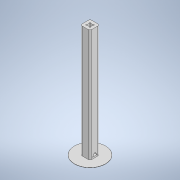
# Autodesk Inventor part: 130mm Rod Template
Saved by Autodesk Inventor 2022 (Build 260153000, 153)
## iProperties
Created: 2022-06-07
Part Number: 130mm Rod Template
Material: Generic
Document SubType Name: Modeling
Designer: Nick
Density: 1 g/cm^3
Appearance: Default
Author: Nick
Autodesk Inventor part; units mm, degrees
ref_plane "YZ Plane" through (0, 0, 0) normal (1, 0, 0) x (0, 1, 0)
ref_plane "XZ Plane" through (0, 0, 0) normal (0, 1, 0) x (-1, 0, 0)
ref_plane "XY Plane" through (0, 0, 0) normal (0, 0, 1) x (1, 0, 0)
sketch "Sketch1" plane through (0, 0, 0) normal (0, 1, 0) x (-1, 0, 0)
  circle A0 centre (0, 0) radius 2
  arc A1 (2.5, 2.1794) -> (2.5, -2.1794) centre (7, 0) ccw
  arc A2 (2.1794, -2.5) -> (-2.1794, -2.5) centre (0, -7) ccw
  arc A3 (-2.5, -2.1794) -> (-2.5, 2.1794) centre (-7, 0) ccw
  arc A4 (-2.1794, 2.5) -> (2.1794, 2.5) centre (0, 7) ccw
  line L0 (2.5, 2.5) -> (-2.5, 2.5)
  line L1 (-2.5, 2.5) -> (-2.5, -2.5)
  line L2 (-2.5, -2.5) -> (2.5, -2.5)
  line L3 (2.5, -2.5) -> (2.5, 2.5)
  line L4 (-5.5, -5.5) -> (-5.5, 5.5)
  line L5 (-5.5, 5.5) -> (5.5, 5.5)
  line L6 (5.5, 5.5) -> (5.5, -5.5)
  line L7 (5.5, -5.5) -> (-5.5, -5.5)
  point P0 (2.5, 0)
  point P1 (0, -2.5)
  dimension "d0" = 4
  dimension "d1" = 5
  dimension "d2" = 5
  dimension "d3" = 3
  constraints: 16 end point, 8 point on circle, 8 point on line, 5 centre point, 4 parallel, 4 tangent, 3 equal radius, 3 horizontal alignment, 3 perpendicular, 3 vertical alignment, 2 midpoint, 1 coincident, 1 horizontal, 3 other
  measures "d0" diameter of A0
  measures "d1" distance of L0.start L0.end
  measures "d2" radius of A4
  measures "d3" distance between parallel lines of L1 L4
extrude "Extrusion1" add sketch "Sketch1" along normal blind 125 contours A1 L3 | A4 L0 | A2 L2 | A3 L1 | L4 L5 L6 L7
sketch "Sketch2" plane through (5.5, 0, -5.5) normal (0, 0, -1) x (-1, 0, 0)
  line L0 (11, 125) -> (11, 0) construction
  line L1 (11, 0) -> (0, 0) construction
  line L2 (0, 0) -> (0, 125) construction
  line L3 (0, 125) -> (11, 125) construction
  line L4 (0, 0) -> (0, 125) projected
  line L5 (0, 125) -> (11, 125) projected
  line L6 (11, 0) -> (11, 125) projected
  line L7 (0, 0) -> (11, 0) projected
  line L8 (2.45, 72.5101) -> (2.45, 75.486)
  line L9 (2.45, 75.486) -> (3.0729, 75.486)
  line L10 (3.0729, 75.486) -> (3.0729, 74.3787)
  line L11 (3.0729, 74.3787) -> (7.1609, 74.3787)
  line L12 (7.1609, 74.3787) -> (7.1609, 75.486)
  line L13 (7.1609, 75.486) -> (7.7195, 75.486)
  spline S0 degree 2 poles (7.7195, 75.486) (7.7195, 74.8582) (8.0754, 74.265) (8.5698, 74.2254) knots 0 0 0 1 2 2 2
  line L14 (8.5698, 74.2254) -> (8.5698, 73.5927)
  line L15 (8.5698, 73.5927) -> (3.0729, 73.5927)
  line L16 (3.0729, 73.5927) -> (3.0729, 72.5101)
  line L17 (3.0729, 72.5101) -> (2.45, 72.5101)
  spline S1 degree 2 poles (7.9716, 69.7419) (7.9716, 69.9643) (7.8629, 70.4043) (7.7788, 70.6169) knots 0 0 0 1 2 2 2
  spline S2 degree 2 poles (7.7788, 70.6169) (7.6948, 70.8146) (7.5169, 71.1062) (7.4378, 71.2199) knots 0 0 0 1 2 2 2
  line L18 (7.4378, 71.2199) -> (7.4378, 71.2694)
  line L19 (7.4378, 71.2694) -> (8.3028, 71.2694)
  spline S3 degree 2 poles (8.3028, 71.2694) (8.4462, 71.0024) (8.6785, 70.0879) (8.6785, 69.6776) knots 0 0 0 1 2 2 2
  spline S4 degree 2 poles (8.6785, 69.6776) (8.6785, 69.2624) (8.5105, 68.6445) (8.3325, 68.3924) knots 0 0 0 1 2 2 2
  spline S5 degree 2 poles (8.3325, 68.3924) (8.1397, 68.1254) (7.5811, 67.8486) (7.2054, 67.8486) knots 0 0 0 1 2 2 2
  spline S6 degree 2 poles (7.2054, 67.8486) (6.7012, 67.8486) (5.94, 68.511) (5.8411, 68.9757) knots 0 0 0 1 2 2 2
  line L20 (5.8411, 68.9757) -> (5.7818, 68.9757)
  spline S7 degree 2 poles (5.7818, 68.9757) (5.7422, 68.7829) (5.5643, 68.343) (5.3863, 68.1551) knots 0 0 0 1 2 2 2
  spline S8 degree 2 poles (5.3863, 68.1551) (5.2133, 67.9673) (4.6596, 67.73) (4.2592, 67.73) knots 0 0 0 1 2 2 2
  spline S9 degree 2 poles (4.2592, 67.73) (3.8489, 67.73) (3.1519, 68.0118) (2.885, 68.2688) knots 0 0 0 1 2 2 2
  spline S10 degree 2 poles (2.885, 68.2688) (2.6082, 68.5357) (2.3215, 69.2921) (2.3215, 69.7716) knots 0 0 0 1 2 2 2
  spline S11 degree 2 poles (2.3215, 69.7716) (2.3215, 70.2313) (2.5439, 71.131) (2.6972, 71.4374) knots 0 0 0 1 2 2 2
  line L21 (2.6972, 71.4374) -> (3.5622, 71.4374)
  line L22 (3.5622, 71.4374) -> (3.5622, 71.3781)
  spline S12 degree 2 poles (3.5622, 71.3781) (3.3744, 71.1211) (3.0284, 70.2511) (3.0284, 69.821) knots 0 0 0 1 2 2 2
  spline S13 degree 2 poles (3.0284, 69.821) (3.0284, 69.5689) (3.1865, 69.0647) (3.3694, 68.8966) knots 0 0 0 1 2 2 2
  spline S14 degree 2 poles (3.3694, 68.8966) (3.5524, 68.7335) (3.9874, 68.5605) (4.3186, 68.5605) knots 0 0 0 1 2 2 2
  spline S15 degree 2 poles (4.3186, 68.5605) (4.6498, 68.5605) (5.0798, 68.7532) (5.2034, 68.9263) knots 0 0 0 1 2 2 2
  spline S16 degree 2 poles (5.2034, 68.9263) (5.327, 69.0993) (5.4209, 69.5689) (5.4209, 69.8457) knots 0 0 0 1 2 2 2
  line L23 (5.4209, 69.8457) -> (5.4209, 70.1917)
  line L24 (5.4209, 70.1917) -> (6.0981, 70.1917)
  line L25 (6.0981, 70.1917) -> (6.0981, 69.9199)
  spline S17 degree 2 poles (6.0981, 69.9199) (6.0981, 69.3712) (6.6221, 68.6791) (7.1214, 68.6791) knots 0 0 0 1 2 2 2
  spline S18 degree 2 poles (7.1214, 68.6791) (7.3537, 68.6791) (7.6849, 68.8571) (7.7838, 69.0004) knots 0 0 0 1 2 2 2
  spline S19 degree 2 poles (7.7838, 69.0004) (7.8876, 69.1536) (7.9716, 69.5293) (7.9716, 69.7419) knots 0 0 0 1 2 2 2
  spline S20 degree 2 poles (5.5, 63.0141) (3.8588, 63.0141) (2.3215, 63.9682) (2.3215, 64.9618) knots 0 0 0 1 2 2 2
  spline S21 degree 2 poles (2.3215, 64.9618) (2.3215, 65.9702) (3.8885, 66.9143) (5.4951, 66.9143) knots 0 0 0 1 2 2 2
  spline S22 degree 2 poles (5.4951, 66.9143) (7.1461, 66.9143) (8.6736, 65.9603) (8.6736, 64.9618) knots 0 0 0 1 2 2 2
  spline S23 degree 2 poles (8.6736, 64.9618) (8.6736, 63.9583) (7.0917, 63.0141) (5.5, 63.0141) knots 0 0 0 1 2 2 2
  spline S24 degree 2 poles (3.6413, 64.0621) (3.9429, 63.9434) (4.8722, 63.8446) (5.5, 63.8446) knots 0 0 0 1 2 2 2
  spline S25 degree 2 poles (5.5, 63.8446) (6.1278, 63.8446) (7.0522, 63.9434) (7.3636, 64.067) knots 0 0 0 1 2 2 2
  spline S26 degree 2 poles (7.3636, 64.067) (7.675, 64.1906) (7.9964, 64.6207) (7.9964, 64.9618) knots 0 0 0 1 2 2 2
  spline S27 degree 2 poles (7.9964, 64.9618) (7.9964, 65.3028) (7.675, 65.7428) (7.3537, 65.8713) knots 0 0 0 1 2 2 2
  spline S28 degree 2 poles (7.3537, 65.8713) (7.0423, 65.9949) (6.0932, 66.0839) (5.4951, 66.0839) knots 0 0 0 1 2 2 2
  spline S29 degree 2 poles (5.4951, 66.0839) (4.8524, 66.0839) (3.9923, 66.0048) (3.6562, 65.8763) knots 0 0 0 1 2 2 2
  spline S30 degree 2 poles (3.6562, 65.8763) (3.3398, 65.7576) (2.9987, 65.3177) (2.9987, 64.9618) knots 0 0 0 1 2 2 2
  spline S31 degree 2 poles (2.9987, 64.9618) (2.9987, 64.6256) (3.32, 64.1857) (3.6413, 64.0621) knots 0 0 0 1 2 2 2
  line L26 (2.45, 56.9289) -> (5.0996, 56.9289)
  spline S32 degree 2 poles (5.0996, 56.9289) (5.416, 56.9289) (5.9548, 56.9784) (6.1031, 57.0575) knots 0 0 0 1 2 2 2
  spline S33 degree 2 poles (6.1031, 57.0575) (6.2662, 57.1365) (6.4244, 57.4381) (6.4244, 57.7001) knots 0 0 0 1 2 2 2
  spline S34 degree 2 poles (6.4244, 57.7001) (6.4244, 57.9374) (6.1327, 58.4811) (5.8559, 58.7678) knots 0 0 0 1 2 2 2
  spline S35 degree 2 poles (5.8559, 58.7678) (5.7867, 58.7629) (5.5939, 58.753) (5.4654, 58.753) knots 0 0 0 1 2 2 2
  line L27 (5.4654, 58.753) -> (2.45, 58.753)
  line L28 (2.45, 58.753) -> (2.45, 59.5241)
  line L29 (2.45, 59.5241) -> (5.0996, 59.5241)
  spline S36 degree 2 poles (5.0996, 59.5241) (5.416, 59.5241) (5.9548, 59.5736) (6.1031, 59.6527) knots 0 0 0 1 2 2 2
  spline S37 degree 2 poles (6.1031, 59.6527) (6.2662, 59.7318) (6.4244, 60.0333) (6.4244, 60.2953) knots 0 0 0 1 2 2 2
  spline S38 degree 2 poles (6.4244, 60.2953) (6.4244, 60.5425) (6.113, 61.0912) (5.8707, 61.3482) knots 0 0 0 1 2 2 2
  line L30 (5.8707, 61.3482) -> (2.45, 61.3482)
  line L31 (2.45, 61.3482) -> (2.45, 62.1194)
  line L32 (2.45, 62.1194) -> (7.0275, 62.1194)
  line L33 (7.0275, 62.1194) -> (7.0275, 61.3482)
  line L34 (7.0275, 61.3482) -> (6.5233, 61.3482)
  spline S39 degree 2 poles (6.5233, 61.3482) (6.8248, 61.0467) (7.156, 60.4535) (7.156, 60.0976) knots 0 0 0 1 2 2 2
  spline S40 degree 2 poles (7.156, 60.0976) (7.156, 59.6922) (6.7853, 59.0644) (6.3651, 58.9013) knots 0 0 0 1 2 2 2
  spline S41 degree 2 poles (6.3651, 58.9013) (6.7556, 58.5503) (7.156, 57.8879) (7.156, 57.5024) knots 0 0 0 1 2 2 2
  spline S42 degree 2 poles (7.156, 57.5024) (7.156, 57.2058) (6.9731, 56.7213) (6.7655, 56.5434) knots 0 0 0 1 2 2 2
  spline S43 degree 2 poles (6.7655, 56.5434) (6.5579, 56.3605) (5.935, 56.1578) (5.4654, 56.1578) knots 0 0 0 1 2 2 2
  line L35 (5.4654, 56.1578) -> (2.45, 56.1578)
  line L36 (2.45, 56.1578) -> (2.45, 56.9289)
  line L37 (2.45, 49.8848) -> (5.0996, 49.8848)
  spline S44 degree 2 poles (5.0996, 49.8848) (5.416, 49.8848) (5.9548, 49.9342) (6.1031, 50.0133) knots 0 0 0 1 2 2 2
  spline S45 degree 2 poles (6.1031, 50.0133) (6.2662, 50.0924) (6.4244, 50.3939) (6.4244, 50.6559) knots 0 0 0 1 2 2 2
  spline S46 degree 2 poles (6.4244, 50.6559) (6.4244, 50.8932) (6.1327, 51.437) (5.8559, 51.7237) knots 0 0 0 1 2 2 2
  spline S47 degree 2 poles (5.8559, 51.7237) (5.7867, 51.7187) (5.5939, 51.7088) (5.4654, 51.7088) knots 0 0 0 1 2 2 2
  line L38 (5.4654, 51.7088) -> (2.45, 51.7088)
  line L39 (2.45, 51.7088) -> (2.45, 52.48)
  line L40 (2.45, 52.48) -> (5.0996, 52.48)
  spline S48 degree 2 poles (5.0996, 52.48) (5.416, 52.48) (5.9548, 52.5294) (6.1031, 52.6085) knots 0 0 0 1 2 2 2
  spline S49 degree 2 poles (6.1031, 52.6085) (6.2662, 52.6876) (6.4244, 52.9891) (6.4244, 53.2511) knots 0 0 0 1 2 2 2
  spline S50 degree 2 poles (6.4244, 53.2511) (6.4244, 53.4983) (6.113, 54.047) (5.8707, 54.3041) knots 0 0 0 1 2 2 2
  line L41 (5.8707, 54.3041) -> (2.45, 54.3041)
  line L42 (2.45, 54.3041) -> (2.45, 55.0752)
  line L43 (2.45, 55.0752) -> (7.0275, 55.0752)
  line L44 (7.0275, 55.0752) -> (7.0275, 54.3041)
  line L45 (7.0275, 54.3041) -> (6.5233, 54.3041)
  spline S51 degree 2 poles (6.5233, 54.3041) (6.8248, 54.0025) (7.156, 53.4093) (7.156, 53.0534) knots 0 0 0 1 2 2 2
  spline S52 degree 2 poles (7.156, 53.0534) (7.156, 52.6481) (6.7853, 52.0203) (6.3651, 51.8571) knots 0 0 0 1 2 2 2
  spline S53 degree 2 poles (6.3651, 51.8571) (6.7556, 51.5062) (7.156, 50.8438) (7.156, 50.4582) knots 0 0 0 1 2 2 2
  spline S54 degree 2 poles (7.156, 50.4582) (7.156, 50.1616) (6.9731, 49.6771) (6.7655, 49.4992) knots 0 0 0 1 2 2 2
  spline S55 degree 2 poles (6.7655, 49.4992) (6.5579, 49.3163) (5.935, 49.1136) (5.4654, 49.1136) knots 0 0 0 1 2 2 2
  line L46 (5.4654, 49.1136) -> (2.45, 49.1136)
  line L47 (2.45, 49.1136) -> (2.45, 49.8848)
  point P0 (5.5, 0)
  constraints: 4 collinear, 1 vertical, 2 other
emboss "Emboss1" sketch "Sketch2" operation cut depth 0.2 direction (0, 0, 1) contours L8 L9 L10 L11 L12 L13 S0 L14 L15 L16 L17 | S1 S2 L18 L19 S3 S4 S5 S6 L20 S7 S8 S9 S10 S11 L21 L22 S12 S13 S14 S15 S16 L23 L24 L25 S17 S18 S19 | S20 S21 S22 S23 | L26 S32 S33 S34 S35 L27 L28 L29 S36 S37 S38 L30 L31 L32 L33 L34 S39 S40 S41 S42 S43 L35 L36 | L37 S44 S45 S46 S47 L38 L39 L40 S48 S49 S50 L41 L42 L43 L44 L45 S51 S52 S53 S54 S55 L46 L47
fillet "Fillet1" radius 2 4 edges at (-5.5, 62.5, 5.5) (-5.5, 62.5, -5.5) (5.5, 62.5, -5.5) (5.5, 62.5, 5.5)
sketch "Sketch3" plane through (0, 0, 0) normal (0, -1, 0) x (1, 0, 0)
  arc A0 (5.5, 3.5) -> (3.5, 5.5) centre (3.5, 3.5) ccw projected
  line L0 (-3.5, 5.5) -> (3.5, 5.5) projected
  arc A1 (-3.5, 5.5) -> (-5.5, 3.5) centre (-3.5, 3.5) ccw projected
  line L1 (-5.5, -3.5) -> (-5.5, 3.5) projected
  arc A2 (-5.5, -3.5) -> (-3.5, -5.5) centre (-3.5, -3.5) ccw projected
  line L2 (3.5, -5.5) -> (-3.5, -5.5) projected
  arc A3 (3.5, -5.5) -> (5.5, -3.5) centre (3.5, -3.5) ccw projected
  line L3 (5.5, 3.5) -> (5.5, -3.5) projected
  arc A4 (-2.5, -2.1794) -> (-2.5, 2.1794) centre (-7, 0) ccw projected
  line L4 (-2.5, 2.5) -> (-2.5, 2.1794) projected
  line L5 (-2.1794, 2.5) -> (-2.5, 2.5) projected
  arc A5 (-2.1794, 2.5) -> (2.1794, 2.5) centre (0, 7) ccw projected
  line L6 (2.5, 2.5) -> (2.1794, 2.5) projected
  line L7 (2.5, 2.1794) -> (2.5, 2.5) projected
  arc A6 (2.5, 2.1794) -> (2.5, -2.1794) centre (7, 0) ccw projected
  line L8 (2.5, -2.5) -> (2.5, -2.1794) projected
  line L9 (2.1794, -2.5) -> (2.5, -2.5) projected
  arc A7 (2.1794, -2.5) -> (-2.1794, -2.5) centre (0, -7) ccw projected
  line L10 (-2.5, -2.5) -> (-2.1794, -2.5) projected
  line L11 (-2.5, -2.1794) -> (-2.5, -2.5) projected
  point P0 (0, 0)
extrude "Extrusion2" add sketch "Sketch3" along normal blind 2 contours L3 A3 L2 A2 L1 A1 L0 A0 | A4 L4 L5 A5 L6 L7 A6 L8 L9 A7 L10 L11
sketch "Sketch4" plane through (5.5, 125, 3.5) normal (1, 0, 0) x (0, 0, -1)
  line L0 (5.6794, -125) -> (1.3206, -125) projected
  line L1 (6, -122) -> (1, -122)
  line L2 (1, -122) -> (1, -125)
  line L3 (1, -125) -> (6, -125)
  line L4 (6, -125) -> (6, -122)
  line L5 (6, -125) -> (4.2679, -122)
  line L6 (1, -125) -> (2.7321, -122)
  point P0 (3.5, -125)
  point P1 (1.3206, -125)
  dimension "d17" = 5
  dimension "d18" = 3
  dimension "d19" = 60
  dimension "d20" = 60
  constraints: 12 end point, 2 midpoint, 2 parallel, 2 point on line, 1 horizontal, 1 perpendicular
  measures "d17" distance of L3.end L2.end
  measures "d18" distance of L2.end L1.end
  measures "d19" angle of L3 L6
  measures "d20" angle of L3 L5
extrude "Extrusion3" cut sketch "Sketch4" against normal through all contours L0 L3 L6 L1 L5
sketch "Sketch5" plane through (0, -2, 0) normal (0, -1, 0) x (1, 0, 0)
  circle A0 centre (0, 0) radius 17.5
  dimension "d21" = 35
  constraints: 1 centre point, 1 coincident
  measures "d21" diameter of A0
extrude "Extrusion4" add sketch "Sketch5" against normal blind 0.2
sketch "Sketch6" plane through (0, -2, 0) normal (0, -1, 0) x (1, 0, 0)
  circle A0 centre (0, 0) radius 0.75
  dimension "d24" = 1.5
  constraints: 1 centre point, 1 coincident
  measures "d24" diameter of A0
extrude "Extrusion5" cut sketch "Sketch6" against normal through all
body "Solid1"
